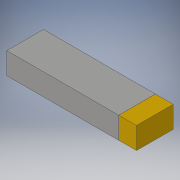
# Autodesk Inventor part: battery
Saved by Autodesk Inventor 2018 (Build 220112000, 112)
## iProperties
Created: 2018-03-12
Part Number: battery
Material: Generic
Document SubType Name: Modeling
Designer: Josh
Density: 1 g/cm^3
Appearance: Galvanized
Author: Josh
Autodesk Inventor part; units mm, degrees
ref_plane "YZ Plane" through (0, 0, 0) normal (1, 0, 0) x (0, 1, 0)
ref_plane "XZ Plane" through (0, 0, 0) normal (0, 1, 0) x (-1, 0, 0)
ref_plane "XY Plane" through (0, 0, 0) normal (0, 0, 1) x (1, 0, 0)
sketch "Sketch1" plane through (0, 0, 0) normal (0, 1, 0) x (-1, 0, 0)
  line L0 (0, 0) -> (127.9906, 0)
  line L1 (127.9906, 0) -> (127.9906, -41.9862)
  line L2 (127.9906, -41.9862) -> (0, -41.9862)
  line L3 (0, -41.9862) -> (0, 0)
  dimension "d0" = 127.9906
  dimension "d1" = 41.9862
  constraints: 8 end point, 2 parallel, 1 horizontal, 1 perpendicular
  measures "d0" distance of L1.end L2.end
  measures "d1" distance of L0.end L1.end
extrude "Extrusion1" add sketch "Sketch1" along normal blind 24.892
sketch "Sketch2" plane through (0, 0, 0) normal (1, 0, 0) x (0, 0, -1)
  line L0 (0.0584, 0.0419) -> (41.946, 0.0419)
  line L1 (41.946, 0.0419) -> (41.946, 24.8567)
  line L2 (41.946, 24.8567) -> (0.0584, 24.8567)
  line L3 (0.0584, 24.8567) -> (0.0584, 0.0419)
  point P0 (0, 0)
  point P1 (41.9862, 24.892)
  constraints: 8 end point, 2 parallel, 1 horizontal, 1 perpendicular
extrude "Extrusion2" add sketch "Sketch2" along normal blind 20.32
body "Solid1"
